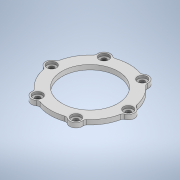
# Autodesk Inventor part: Outer_flange
Saved by Autodesk Inventor 2020.4 (Build 244396000, 396)
## iProperties
Created: 2021-12-30
Part Number: Outer_flange
Material: アルミニウム 2014-T4
Document SubType Name: Modeling
Designer: Masato Kubotera
Density: 2.8 g/cm^3
Appearance: 滑らか - 淡い灰色
Author: Masato Kubotera
Autodesk Inventor part; units mm, degrees
ref_plane "YZ Plane" through (0, 0, 0) normal (1, 0, 0) x (0, 1, 0)
ref_plane "XZ Plane" through (0, 0, 0) normal (0, 1, 0) x (-1, 0, 0)
ref_plane "XY Plane" through (0, 0, 0) normal (0, 0, 1) x (1, 0, 0)
derived "Outer_support_stand.ipt"
sketch "スケッチ1" plane through (0, 0, 0) normal (0, 0, 1) x (1, 0, 0)
  circle A0 centre (0, 0) radius 18.5
  circle A1 centre (0, 0) radius 20.5 construction
  circle A2 centre (0, 0) radius 20.51
  line L0 (0, 0) -> (0, 24.5) construction
  circle A3 centre (0, 24.5) radius 1.55
  circle A4 centre (0, 24.5) radius 3 construction
  arc A5 (0, 28.5) -> (-3.7147, 25.9835) centre (0, 24.5) ccw
  arc A6 (-5.1639, 24.7674) -> (-18.8673, 16.8557) centre (0, 0) ccw
  arc A7 (-5.1639, 24.7674) -> (-3.7147, 25.9835) centre (-5.5721, 26.7253) ccw
  arc A8 (3.7147, 25.9835) -> (5.1639, 24.7674) centre (5.5721, 26.7253) ccw
  arc A9 (3.7147, 25.9835) -> (0, 28.5) centre (0, 24.5) ccw
  circle A10 centre (0, 24.5) radius 3.05
  arc A11 (-24.0311, 7.9117) -> (-24.0311, -7.9117) centre (0, 0) ccw
  arc A12 (-24.0311, 7.9117) -> (-24.3598, 9.7747) centre (-25.9308, 8.5371) ccw
  arc A13 (-24.6817, 14.25) -> (-24.3598, 9.7747) centre (-21.2176, 12.25) ccw
  arc A14 (-20.645, 16.2088) -> (-24.6817, 14.25) centre (-21.2176, 12.25) ccw
  arc A15 (-20.645, 16.2088) -> (-18.8673, 16.8557) centre (-20.3588, 18.1882) ccw
  circle A16 centre (-21.2176, 12.25) radius 3.05
  circle A17 centre (-21.2176, 12.25) radius 1.55
  arc A18 (-18.8673, -16.8557) -> (-5.1639, -24.7674) centre (0, 0) ccw
  arc A19 (-18.8673, -16.8557) -> (-20.645, -16.2088) centre (-20.3588, -18.1882) ccw
  arc A20 (-24.6817, -14.25) -> (-20.645, -16.2088) centre (-21.2176, -12.25) ccw
  arc A21 (-24.3598, -9.7747) -> (-24.6817, -14.25) centre (-21.2176, -12.25) ccw
  arc A22 (-24.3598, -9.7747) -> (-24.0311, -7.9117) centre (-25.9308, -8.5371) ccw
  circle A23 centre (-21.2176, -12.25) radius 3.05
  circle A24 centre (-21.2176, -12.25) radius 1.55
  arc A25 (5.1639, -24.7674) -> (18.8673, -16.8557) centre (0, 0) ccw
  arc A26 (5.1639, -24.7674) -> (3.7147, -25.9835) centre (5.5721, -26.7253) ccw
  arc A27 (0, -28.5) -> (3.7147, -25.9835) centre (0, -24.5) ccw
  arc A28 (-3.7147, -25.9835) -> (0, -28.5) centre (0, -24.5) ccw
  arc A29 (-3.7147, -25.9835) -> (-5.1639, -24.7674) centre (-5.5721, -26.7253) ccw
  circle A30 centre (0, -24.5) radius 3.05
  circle A31 centre (0, -24.5) radius 1.55
  arc A32 (24.0311, -7.9117) -> (24.0311, 7.9117) centre (0, 0) ccw
  arc A33 (24.0311, -7.9117) -> (24.3598, -9.7747) centre (25.9308, -8.5371) ccw
  arc A34 (24.6817, -14.25) -> (24.3598, -9.7747) centre (21.2176, -12.25) ccw
  arc A35 (20.645, -16.2088) -> (24.6817, -14.25) centre (21.2176, -12.25) ccw
  arc A36 (20.645, -16.2088) -> (18.8673, -16.8557) centre (20.3588, -18.1882) ccw
  circle A37 centre (21.2176, -12.25) radius 3.05
  circle A38 centre (21.2176, -12.25) radius 1.55
  arc A39 (18.8673, 16.8557) -> (5.1639, 24.7674) centre (0, 0) ccw
  arc A40 (18.8673, 16.8557) -> (20.645, 16.2088) centre (20.3588, 18.1882) ccw
  arc A41 (24.6817, 14.25) -> (20.645, 16.2088) centre (21.2176, 12.25) ccw
  arc A42 (24.3598, 9.7747) -> (24.6817, 14.25) centre (21.2176, 12.25) ccw
  arc A43 (24.3598, 9.7747) -> (24.0311, 7.9117) centre (25.9308, 8.5371) ccw
  circle A44 centre (21.2176, 12.25) radius 3.05
  circle A45 centre (21.2176, 12.25) radius 1.55
  circle A46 centre (0, 0) radius 17.9
  point P0 (-24.0311, -7.9117)
  point P1 (18.8673, -16.8557)
  point P2 (24.0311, 7.9117)
  dimension "d5" = 35.8
  measures "d5" diameter of A46
extrude "押し出し1" add sketch "スケッチ1" along normal blind 3 contours A0 | A2 | A9 A8 A39 A40 A41 A42 A43 A32 A33 A34 A35 A36 A25 A26 A27 A28 A29 A18 A19 A20 A21 A22 A11 A12 A13 A14 A15 A6 A7 A5
extrude "押し出し2" add sketch "スケッチ1" along normal blind 1.5 contours A10 | A16 | A23 | A30 | A37 | A44
